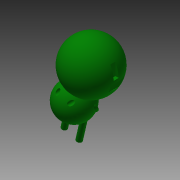
# Autodesk Inventor part: Guisante
Saved by Autodesk Inventor 2014 (Build 180170000, 170)
## iProperties
Created: 2015-01-02
Part Number: Guisante
Material: Generic
Document SubType Name: Modeling
Designer: Rubén
Density: 1 g/cm^3
Appearance: Dark Green
Author: Rubén
Autodesk Inventor part; units mm, degrees
ref_plane "YZ Plane" through (0, 0, 0) normal (1, 0, 0) x (0, 1, 0)
ref_plane "XZ Plane" through (0, 0, 0) normal (0, 1, 0) x (-1, 0, 0)
ref_plane "XY Plane" through (0, 0, 0) normal (0, 0, 1) x (1, 0, 0)
sketch "Sketch1" plane through (0, 0, 0) normal (0, 1, 0) x (-1, 0, 0)
  line L0 (0, 0) -> (15, 0)
  line L1 (15, 0) -> (15, 30)
  line L2 (15, 30) -> (0, 30)
  line L3 (0, 30) -> (0, 0)
  dimension "d0" = 15
  dimension "d1" = 30
  constraints: 8 end point, 2 parallel, 1 horizontal, 1 perpendicular
  measures "d0" distance of L0.start L0.end
  measures "d1" distance of L0.end L1.end
extrude "Extrusion1" add sketch "Sketch1" along normal blind 30
sketch "Sketch2" plane through (0, 0, 30) normal (1, 0, 0) x (0, 0, -1)
  line L0 (0, 30) -> (30, 30) projected
  line L1 (16.5, 15) -> (16.5, 30)
  line L2 (13.5, 15) -> (13.5, 30)
  line L3 (13.5, 15) -> (16.5, 15)
  constraints: 6 end point, 3 perpendicular, 2 point on line
extrude "Extrusion3" cut sketch "Sketch2" against normal blind 2
sketch "Sketch7" plane through (-15, 0, 0) normal (-1, 0, 0) x (0, 0, 1)
  line L0 (0, 0) -> (30, 0) projected
  line L1 (0, 30) -> (30, 30) projected
  line L2 (15, 30) -> (15, 0) construction
  arc A0 (15, 30) -> (15, 0) centre (15, 15) ccw
  line L3 (15, 30) -> (15, 0)
  constraints: 4 end point, 3 midpoint, 2 point on circle, 1 centre point, 1 perpendicular
revolve "Revolution2" cut sketch "Sketch7" angle 360 about axis through (-15, 30, 15) along (0, -1, 0) keep common part
mirror "Mirror2" about plane through (-15, 0, 0) normal (-1, 0, 0)
ref_plane "Work Plane3" through (-15, 15, 0) normal (0, 0, -1) x (-1, 0, 0)
sketch "Sketch8" plane through (-15, 15, 0) normal (0, 0, -1) x (-1, 0, 0)
  ellipse E0 centre (2.385555, -11.268925) end of major axis (2.88297, -10.416213) minor radius 0.736313
  point P0 (-15, -15)
  constraints: 2 other
extrude "Extrusion4" cut sketch "Sketch8" against normal blind 6.6
ref_plane "Work Plane4" through (-15, 0, 15) normal (0, 1, 0) x (-1, 0, 0)
sketch "Sketch10" plane through (-15, 15, 0) normal (0, 0, -1) x (-1, 0, 0)
  line L0 (0, 0) -> (0, -11.011003) construction
  line L1 (-7, -1) -> (-4, -1)
  line L2 (-4, -1) -> (-4, -4)
  line L3 (-4, -4) -> (-7, -4)
  line L4 (-7, -4) -> (-7, -1)
  line L5 (7, -1) -> (4, -1)
  line L6 (4, -1) -> (4, -4)
  line L7 (4, -4) -> (7, -4)
  line L8 (7, -4) -> (7, -1)
  point P0 (-15, -15)
  constraints: 18 end point, 4 symmetric about line, 2 parallel, 1 horizontal, 1 perpendicular, 1 vertical
extrude "Extrusion6" cut sketch "Sketch10" against normal blind 8
sketch "Sketch13" plane through (-15, 15, 0) normal (0, 0, -1) x (-1, 0, 0)
  line L0 (-15.727491, -2.5) -> (15.78201, -2.5) construction
  line L1 (-13.5, -1.9) -> (-13.5, -4)
  line L2 (-13.5, -1.9) -> (-17, -1.9)
  line L3 (-17, -1.9) -> (-17, -4)
  line L4 (-17, -4) -> (-13.5, -4)
  line L5 (0, 4.018865) -> (0, -10.79124) construction
  line L6 (13.5, -1.9) -> (13.5, -4)
  line L7 (13.5, -1.9) -> (17, -1.9)
  line L8 (17, -1.9) -> (17, -4)
  line L9 (17, -4) -> (13.5, -4)
  point P0 (-15, -15)
  dimension "d39" = 3.5
  dimension "d40" = 2.1
  dimension "d89" = 13.5
  dimension "d96" = 1.5
  dimension "d97" = 1.5
  dimension "d98" = 11
  constraints: 20 end point, 4 perpendicular, 4 symmetric about line, 1 horizontal
  measures "d39" distance of L1.start L2.end
  measures "d40" distance of L2.end L3.end
  measures "d89" distance from line of L5 L1.start
  measures "d96" distance between parallel lines of L4 L0
  measures "d97" distance from line of L1 point (-15, -15)
  measures "d98" vertical distance of L1.end point (-15, -15)
extrude "Extrusion7" cut sketch "Sketch13" against normal blind 18
ref_plane "Work Plane5" through (-15, 11, 15) normal (0, 0, 1) x (0, -1, 0)
ref_plane "Work Plane6" through (-15, 11, 21) normal (0, 0, 1) x (0, -1, 0)
sketch "Sketch16" plane through (-15, 11, 21) normal (0, 0, 1) x (0, -1, 0)
  line L0 (3.441525, -1.960015) -> (33.360723, -8.262418) construction
  arc A0 (23.503378, -6.185993) -> (3.345745, -1.93984) centre (13.424561, -4.062916) ccw
  line L1 (23.503378, -6.185993) -> (3.345745, -1.93984)
  point P0 (11, 15)
  dimension "d48" = 10.3
  constraints: 4 end point, 2 point on circle, 2 point on line, 1 centre point, 1 collinear
  measures "d48" radius of A0
revolve "Revolution3" add sketch "Sketch16" angle 360 about axis through (-16.960015, 7.558475, 21) along (-0.206124, -0.9785259, 0)
ref_plane "Work Plane11" through (-15, 15, 15) normal (-0.973876, 0.2270804, 0) x (-0.2152971, -0.9233409, 0.3179446)
ref_plane "Work Plane12" through (-19.062916, -2.424561, 21) normal (-0.2270804, -0.973876, 0) x (0, 0, 1)
sketch "Sketch21" plane through (-19.062916, -2.424561, 21) normal (-0.2270804, -0.973876, 0) x (0, 0, 1)
  circle A0 centre (-3.396254, 4.431929) radius 1.6
  circle A1 centre (-3.500778, -4.567464) radius 1.6
  point P0 (-21, -18.014347)
  dimension "d58" = 3.2
  dimension "d59" = 3.2
  dimension "d62" = 9
  constraints: 2 centre point
  measures "d58" diameter of A0
  measures "d59" diameter of A1
  measures "d62" distance of A1.centre A0.centre
extrude "Extrusion9" add sketch "Sketch21" along normal blind 22
fillet "Fillet1" radius 2 2 edges at (-16.3324, -10.9462, 15.8994) (-25.1794, -9.0365, 16.0039)
ref_plane "Work Plane14" through (-28.356051, 1.757391, 18.101909) normal (-0.1273217, -0.5460423, 0.828026) x (0.973876, -0.2270804, 0)
ref_plane "Work Plane13" through (-28.801677, -0.153757, 21) normal (-0.1273217, -0.5460423, 0.828026) x (0.973876, -0.2270804, 0)
sketch "Sketch22" plane through (-28.356051, 1.757391, 18.101909) normal (-0.1273217, -0.5460423, 0.828026) x (0.973876, -0.2270804, 0)
  line L0 (2.187892, 1.285581) -> (-1.738355, -0.056741) construction
  line L1 (-1.738355, -0.056741) -> (1.375187, -6.234959) construction
  line L2 (1.375187, -6.234959) -> (4.329603, -8.741292) construction
  line L3 (4.329603, -8.741292) -> (6.997644, -9.253261) construction
  spline S0 degree 4 poles (2.187892, 1.285581) (-1.738355, -0.056741) (1.375187, -6.234959) (4.329603, -8.741292) (6.997644, -9.253261) knots 1 1 1 1 1 2 2 2 2 2
  point P0 (28.014347, -6.234959)
  constraints: 3 other
ref_plane "Work Plane16" through (-25.983589, 2.297249, 18.822721) normal (-0.982336, -0.0459993, -0.1813835) x (0.0467752, -0.9989054, 0)
sketch "Sketch25" plane through (-25.983589, 2.297249, 18.822721) normal (-0.982336, -0.0459993, -0.1813835) x (0.0467752, -0.9989054, 0)
  circle A0 centre (0, 0) radius 1
  point P0 (3.510122, -23.198843)
  dimension "d72" = 2
  constraints: 1 centre point
  measures "d72" diameter of A0
sweep "Sweep2" add profiles "Sketch25" path "Sketch22"
sketch "Sketch26" plane through (-28.356051, 1.757391, 18.101909) normal (-0.1273217, -0.5460423, 0.828026) x (0.973876, -0.2270804, 0)
  line L0 (18.329628, 1.837089) -> (21.387938, -0.778644) construction
  line L1 (21.387938, -0.778644) -> (17.958311, -6.628325) construction
  line L2 (17.958311, -6.628325) -> (15.305664, -8.445264) construction
  line L3 (15.305664, -8.445264) -> (12.33985, -8.568624) construction
  spline S0 degree 4 poles (18.329628, 1.837089) (21.387938, -0.778644) (17.958311, -6.628325) (15.305664, -8.445264) (12.33985, -8.568624) knots 1 1 1 1 1 2 2 2 2 2
  point P0 (28.014347, -6.234959)
  constraints: 3 other
ref_plane "Work Plane17" through (-10.159841, -0.92349, 19.131946) normal (0.6178855, -0.6967093, -0.364436) x (0.7481615, 0.6635166, 0)
sketch "Sketch27" plane through (-10.159841, -0.92349, 19.131946) normal (0.6178855, -0.6967093, -0.364436) x (0.7481615, 0.6635166, 0)
  circle A0 centre (0, 0) radius 1
  point P0 (8.213953, -15.611263)
  dimension "d75" = 2
  constraints: 1 centre point
  measures "d75" diameter of A0
sweep "Sweep3" add profiles "Sketch27" path "Sketch26"
ref_plane "Work Plane18" through (-17.60956, -2.711087, 21.034526) normal (-0.9808488, 0.1933721, -0.0233012) x (0.0889353, 0.5510876, 0.8296945)
ref_plane "Work Plane19" through (-22.820594, -7.480906, 12.860869) normal (0.9209924, -0.3749779, -0.1056627) x (-0.3027399, -0.5181658, -0.799908)
sketch "Sketch29" plane through (-17.60956, -2.711087, 21.034526) normal (-0.9808488, 0.1933721, -0.0233012) x (0.0889353, 0.5510876, 0.8296945)
  arc A0 (-10.155088, 1.398904) -> (-10.247724, -1.372983) centre (-10.201406, 0.012961) ccw
  line L0 (-10.155088, 1.398904) -> (-10.247724, -1.372983) construction
  line L1 (-10.155088, 1.398904) -> (-10.247724, -1.372983)
  point P0 (-14.392072, 16.983686)
  constraints: 4 end point, 2 point on circle, 1 centre point, 1 collinear
revolve "Revolution4" add sketch "Sketch29" angle 360 about axis through (-18.270303, -7.171894, 11.828693) along (-0.1761546, -0.8296865, 0.5297074)
sketch "Sketch30" plane through (-22.820594, -7.480906, 12.860869) normal (0.9209924, -0.3749779, -0.1056627) x (-0.3027399, -0.5181658, -0.799908)
  arc A0 (0.253581, -1.325621) -> (0.167759, 1.320564) centre (0.21067, -0.002528) ccw
  line L0 (0.167759, 1.320564) -> (0.253581, -1.325621)
  line L1 (0.167759, 1.320564) -> (0.253581, -1.325621) construction
  point P0 (-0.497542, 18.943621)
  constraints: 4 end point, 2 point on circle, 1 centre point, 1 collinear
revolve "Revolution5" add sketch "Sketch30" angle 360 about axis through (-22.547583, -6.552719, 11.946558) along (-0.2548816, -0.7850901, 0.5645077)
ref_plane "Work Plane20" through (-19.062916, -2.424561, 21) normal (0, 0, 1) x (-0.973876, 0.2270804, 0)
sketch "Sketch31" plane through (-19.062916, -2.424561, 21) normal (0, 0, 1) x (-0.973876, 0.2270804, 0)
  line L0 (0, 0) -> (0, -10.30348) construction
  circle A0 centre (4, -6) radius 1.25
  circle A1 centre (-4, -6) radius 1.25
  point P0 (-18.014347, -6.690037)
  dimension "d85" = 2.5
  constraints: 2 centre point, 2 end point, 1 symmetric about line, 1 other
  measures "d85" diameter of A0
extrude "Extrusion10" cut sketch "Sketch31" along normal blind 10
sketch "Sketch32" plane through (-15, 15, 0) normal (0, 0, -1) x (-1, 0, 0)
  line L0 (-13.5, -4) -> (-13.5, -5.93)
  line L1 (-13.5, -5.93) -> (-15.5, -5.93)
  line L2 (-15.5, -5.93) -> (-15.5, -4)
  line L3 (-15.5, -4) -> (-13.5, -4)
  line L4 (0, 0) -> (0, -11.735573) construction
  line L5 (13.5, -4) -> (13.5, -5.93)
  line L6 (13.5, -5.93) -> (15.5, -5.93)
  line L7 (15.5, -5.93) -> (15.5, -4)
  line L8 (15.5, -4) -> (13.5, -4)
  point P0 (-15, -15)
  dimension "d90" = 1.93
  dimension "d91" = 2
  dimension "d94" = 11
  dimension "d95" = 1.5
  constraints: 18 end point, 4 symmetric about line, 2 parallel, 2 perpendicular, 1 vertical
  measures "d90" distance of L0.start L0.end
  measures "d91" distance of L0.end L1.end
  measures "d94" distance from line of L3 point (-15, -15)
  measures "d95" distance from line of L0 point (-15, -15)
extrude "Extrusion11" cut sketch "Sketch32" against normal up to surface (18 mm away)
body "Solid1"
